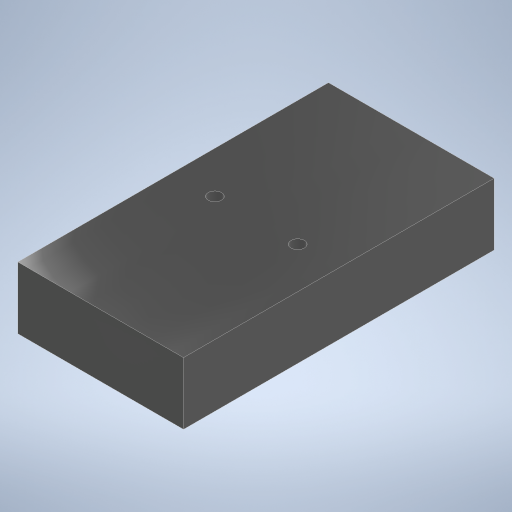
# Autodesk Inventor part: холдер
Saved by Autodesk Inventor 2023.1 (Build 271208000, 208)
## iProperties
Created: 2026-02-22
Part Number: холдер
Material: Типовые
Document SubType Name: Modeling
Designer: DELL
Density: 1 g/cm^3
Appearance: Темно-серый
Author: DELL
Autodesk Inventor part; units mm, degrees
ref_plane "YZ Plane" through (0, 0, 0) normal (1, 0, 0) x (0, 1, 0)
ref_plane "XZ Plane" through (0, 0, 0) normal (0, 1, 0) x (-1, 0, 0)
ref_plane "XY Plane" through (0, 0, 0) normal (0, 0, 1) x (1, 0, 0)
sketch "Эскиз1" plane through (0, 0, 0) normal (0, 1, 0) x (-1, 0, 0)
  line L0 (-20, 37.5) -> (20, 37.5)
  line L1 (20, 37.5) -> (20, -37.5)
  line L2 (20, -37.5) -> (-20, -37.5)
  line L3 (-20, -37.5) -> (-20, 37.5)
  line L4 (-20, 37.5) -> (20, -37.5) construction
  line L5 (20, 37.5) -> (-20, -37.5) construction
  point P0 (0, 0)
  dimension "d0" = 75
  dimension "d1" = 40
  constraints: 12 end point, 2 midpoint, 2 parallel, 1 horizontal, 1 perpendicular
  measures "d0" distance of L0.end L1.end
  measures "d1" distance of L1.end L2.end
extrude "Выдавливание1" add sketch "Эскиз1" along normal blind 15
sketch "Эскиз2" plane through (0, 15, 0) normal (0, 1, 0) x (1, 0, 0)
  circle A0 centre (10.0691, 0) radius 1.6
  circle A1 centre (-9.9309, 0) radius 1.6
  line L0 (-9.9309, 0) -> (10.0691, 0)
  line L1 (20, 37.5) -> (-20, 37.5) projected
  line L2 (0, 37.5) -> (0, -37.5)
  line L3 (-20, -37.5) -> (20, -37.5) projected
  line L4 (-20, 37.5) -> (-20, -37.5) projected
  line L5 (-20, 0) -> (20.2069, 0)
  point P0 (0, 0)
  point P1 (0.0691, 0)
  dimension "d4" = 3.2
  dimension "d5" = 3.2
  dimension "d6" = 20
  constraints: 6 end point, 4 midpoint, 2 centre point, 1 horizontal, 1 perpendicular, 1 point on line
  measures "d4" diameter of A0
  measures "d5" diameter of A1
  measures "d6" distance of L0.end L0.start
extrude "Выдавливание2" cut sketch "Эскиз2" against normal blind 15 contours L5 L0 A0 | A0 L0 L5 | L0 L5 A1 | A1 L5 L0
